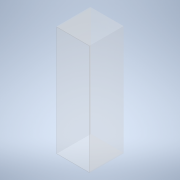
# Autodesk Inventor part: uv environment
Saved by Autodesk Inventor 2021 (Build 250183000, 183)
## iProperties
Created: 2021-07-27
Part Number: uv environment
Material: PMMA Plastic
Document SubType Name: Modeling
Designer: HP
Density: 1.188 g/cm^3
Appearance: Polycarbonate - Clear
Author: HP
Autodesk Inventor part; units mm, degrees
ref_plane "YZ Plane" through (0, 0, 0) normal (1, 0, 0) x (0, 1, 0)
ref_plane "XZ Plane" through (0, 0, 0) normal (0, 1, 0) x (-1, 0, 0)
ref_plane "XY Plane" through (0, 0, 0) normal (0, 0, 1) x (1, 0, 0)
sketch "Sketch1" plane through (0, 0, 0) normal (0, 0, 1) x (1, 0, 0)
  line L0 (147.6375, 0) -> (-128.5875, 0)
  line L1 (-128.5875, 0) -> (-128.5875, 917.575)
  line L2 (-128.5875, 917.575) -> (147.6375, 917.575)
  line L3 (147.6375, 917.575) -> (147.6375, 0)
  line L4 (142.875, 912.8125) -> (-123.825, 912.8125)
  line L5 (-123.825, 912.8125) -> (-123.825, 4.7625)
  line L6 (-123.825, 4.7625) -> (142.875, 4.7625)
  line L7 (142.875, 4.7625) -> (142.875, 912.8125)
  point P0 (0, 0)
  constraints: 16 end point, 4 parallel, 2 horizontal, 2 perpendicular
extrude "Extrusion1" add sketch "Sketch1" against normal blind 281.94
body "Solid1"
